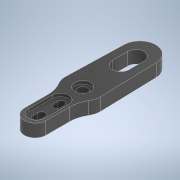
# Autodesk Inventor part: Servo steering actuator v2
Saved by Autodesk Inventor 2022.6 (Build 266554000, 554)
## iProperties
Created: 2024-11-03
Part Number: Servo steering actuator v2
Material: Generic
Document SubType Name: Modeling
Designer: Zhong
Density: 1 g/cm^3
Appearance: Dark Gray
Author: Zhong
Autodesk Inventor part; units mm, degrees
ref_plane "YZ Plane" through (0, 0, 0) normal (1, 0, 0) x (0, 1, 0)
ref_plane "XZ Plane" through (0, 0, 0) normal (0, 1, 0) x (-1, 0, 0)
ref_plane "XY Plane" through (0, 0, 0) normal (0, 0, 1) x (1, 0, 0)
sketch "Sketch1" plane through (0, 0, 0) normal (0, 1, 0) x (-1, 0, 0)
  circle A0 centre (0, 0) radius 1.5
  circle A1 centre (0, 0) radius 5.5
  circle A2 centre (0, -18) radius 5
  line L0 (5.4979, -0.1528) -> (4.9981, -18.1389)
  line L1 (-4.9981, -18.1389) -> (-5.4979, -0.1528)
  line L2 (0, 0) -> (0, 15) construction
  line L3 (-3.4, 0) -> (-3.4, 15)
  line L4 (3.4, 15) -> (3.4, 0)
  arc A3 (-3.4, 0) -> (3.4, 0) centre (0, 0) ccw
  arc A4 (3.4, 15) -> (-3.4, 15) centre (0, 15) ccw
  arc A5 (3.4, 7.5) -> (4.7003, 2.8561) centre (12.3429, 7.5) ccw
  arc A6 (-4.7003, 2.8561) -> (-3.4, 7.5) centre (-12.3429, 7.5) ccw
  point P0 (0, 7.5)
  point P1 (-3.4, 4.3232)
  point P2 (3.4, 4.3232)
  point P3 (-3.4, 7.5)
  dimension "d0" = 3
  dimension "d1" = 11
  dimension "d3" = 18
  dimension "d43" = 15
  dimension "d44" = 3.4
  dimension "d74" = 10
  constraints: 13 point on circle, 12 end point, 10 tangent, 7 centre point, 3 symmetric about line, 2 coincident, 2 midpoint, 1 parallel, 1 vertical, 1 vertical alignment, 1 other
  measures "d0" diameter of A0
  measures "d1" diameter of A1
  measures "d3" distance of point (0, 0) A2.centre
  measures "d43" distance of L2.start L2.end
  measures "d44" radius of A4
  measures "d74" diameter of A2
extrude "Extrusion1" add sketch "Sketch1" along normal blind 4
sketch "Sketch2" plane through (0, 4, 0) normal (0, 1, 0) x (1, 0, 0)
  arc A0 (4.9981, 18.1389) -> (-4.9981, 18.1389) centre (0, 18) ccw projected
  circle A1 centre (0, 0) radius 1.5 projected
  line L0 (0, 16.8) -> (0, 12) construction
  line L1 (-2.6, 16.8) -> (-2.6, 12)
  line L2 (2.6, 12) -> (2.6, 16.8)
  arc A2 (2.6, 16.8) -> (-2.6, 16.8) centre (0, 16.8) ccw
  arc A3 (-2.6, 12) -> (2.6, 12) centre (0, 12) ccw
  line L3 (-3.4, -7.5) -> (-3.4, -15) projected
  arc A4 (-3.4, -15) -> (3.4, -15) centre (0, -15) ccw projected
  line L4 (3.4, -15) -> (3.4, -7.5) projected
  line L5 (-4.9981, 18.1389) -> (-5.4979, 0.1528) projected
  arc A5 (-5.4979, 0.1528) -> (-4.7003, -2.8561) centre (0, 0) ccw projected
  arc A6 (4.7003, -2.8561) -> (5.4979, 0.1528) centre (0, 0) ccw projected
  line L6 (5.4979, 0.1528) -> (4.9981, 18.1389) projected
  arc A7 (-3.4, -7.5) -> (-4.7003, -2.8561) centre (-12.3429, -7.5) ccw projected
  arc A8 (4.7003, -2.8561) -> (3.4, -7.5) centre (12.3429, -7.5) ccw projected
  point P0 (0, 14.4)
  dimension "d6" = 4.8
  dimension "d7" = 5.2
  dimension "d9" = 12
  constraints: 8 end point, 4 point on circle, 4 tangent, 2 centre point, 1 midpoint, 1 parallel, 1 vertical, 1 vertical alignment
  measures "d6" distance of L0.start L0.end
  measures "d7" diameter of A3
  measures "d9" distance of point (0, 0) L0.end
extrude "Extrusion2" cut sketch "Sketch2" against normal through all contours A2 L2 A3 L1
sketch "Sketch8" plane through (0, 4, 0) normal (0, 1, 0) x (1, 0, 0)
  line L0 (0, 31.28) -> (0, -26.68) projected
  line L1 (0, -14.5) -> (0, -7) construction
  line L2 (2.6, -14.5) -> (2.6, -7)
  line L3 (-2.6, -7) -> (-2.6, -14.5)
  arc A0 (-2.6, -14.5) -> (2.6, -14.5) centre (0, -14.5) ccw
  arc A1 (2.6, -7) -> (-2.6, -7) centre (0, -7) ccw
  point P0 (0, 0)
  point P1 (0, -10.75)
  dimension "d45" = 5.2
  dimension "d47" = 7
  dimension "d48" = 14.5
  constraints: 8 end point, 4 point on circle, 4 tangent, 2 centre point, 2 point on line, 1 midpoint, 1 parallel
  measures "d45" diameter of A1
  measures "d47" distance of point (0, 0) L1.end
  measures "d48" distance of point (0, 0) L1.start
extrude "Extrusion8" cut sketch "Sketch8" against normal blind 1
sketch "Sketch10" plane through (0, 0, 0) normal (0, -1, 0) x (1, 0, 0)
  line L0 (0, 6.8) -> (0, 8.2) construction
  line L1 (1.1, 6.8) -> (1.1, 8.2)
  line L2 (-1.1, 8.2) -> (-1.1, 6.8)
  arc A0 (-1.1, 6.8) -> (1.1, 6.8) centre (0, 6.8) ccw
  arc A1 (1.1, 8.2) -> (-1.1, 8.2) centre (0, 8.2) ccw
  line L3 (0, 13) -> (0, 14.5) construction
  line L4 (1.1, 13) -> (1.1, 14.5)
  line L5 (-1.1, 14.5) -> (-1.1, 13)
  arc A2 (-1.1, 13) -> (1.1, 13) centre (0, 13) ccw
  arc A3 (1.1, 14.5) -> (-1.1, 14.5) centre (0, 14.5) ccw
  line L6 (0, -7.3) -> (0, -7.7) construction
  line L7 (1.1, -7.3) -> (1.1, -7.7)
  line L8 (-1.1, -7.7) -> (-1.1, -7.3)
  arc A4 (1.1, -7.3) -> (-1.1, -7.3) centre (0, -7.3) ccw
  arc A5 (-1.1, -7.7) -> (1.1, -7.7) centre (0, -7.7) ccw
  point P0 (0, 0)
  point P1 (0, 7.5)
  point P2 (0, 13.75)
  point P3 (0, -7.5)
  dimension "d60" = 2.2
  dimension "d61" = 6.8
  dimension "d62" = 1.4
  dimension "d63" = 1.5
  dimension "d64" = 2.2
  dimension "d65" = 13
  dimension "d78" = 0.2
  dimension "d79" = 7.5
  constraints: 24 end point, 12 point on circle, 12 tangent, 6 centre point, 3 midpoint, 3 parallel, 3 vertical, 3 vertical alignment, 1 equal radius
  measures "d60" diameter of A1
  measures "d61" distance of point (0, 0) L0.start
  measures "d62" distance of L0.end L0.start
  measures "d63" distance of L3.start L3.end
  measures "d64" diameter of A3
  measures "d65" distance of point (0, 0) L3.start
  measures "d78" distance of point (0, -7.5) L6.end
  measures "d79" distance of point (0, 0) point (0, -7.5)
extrude "Extrusion9" cut sketch "Sketch10" against normal through all contours A0 L2 A1 L1 | A2 L5 A3 L4
sketch "Sketch11" plane through (0, 0, 0) normal (0, -1, 0) x (1, 0, 0)
  circle A0 centre (0, 0) radius 4.25
  dimension "d73" = 8.5
  constraints: 1 centre point, 1 coincident
  measures "d73" diameter of A0
extrude "Extrusion10" cut sketch "Sketch11" against normal blind 0.4
sketch "Sketch12" plane through (0, 4, 0) normal (0, 1, 0) x (1, 0, 0)
  circle A0 centre (0, 0) radius 2.5
  dimension "d75" = 5
  constraints: 1 centre point, 1 coincident
  measures "d75" diameter of A0
extrude "Extrusion11" cut sketch "Sketch12" against normal blind 1
body "Solid1"
